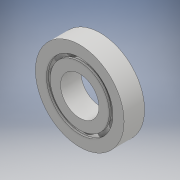
# Autodesk Inventor part: Подшипник 1
Saved by Autodesk Inventor 2018.1 (Build 221171000, 171)
## iProperties
Created: 2018-06-08
Part Number: Подшипник 1
Material: Типовые
Document SubType Name: Modeling
Designer: Dmitry
Density: 1 g/cm^3
Appearance: По умолчанию
Author: Dmitry
Autodesk Inventor part; units mm, degrees
ref_plane "YZ Plane" through (0, 0, 0) normal (1, 0, 0) x (0, 1, 0)
ref_plane "XZ Plane" through (0, 0, 0) normal (0, 1, 0) x (-1, 0, 0)
ref_plane "XY Plane" through (0, 0, 0) normal (0, 0, 1) x (1, 0, 0)
sketch "Эскиз1" plane through (0, 0, 0) normal (0, 0, 1) x (1, 0, 0)
  line L0 (26, 0) -> (26, 27.7778)
  line L1 (26, 27.7778) -> (40, 27.7778)
  line L2 (40, 27.7778) -> (40, 25)
  line L3 (40, 2.7778) -> (40, 0)
  line L4 (40, 0) -> (26, 0)
  arc A0 (40, 25) -> (40, 2.7778) centre (46.2467, 13.8889) ccw
  line L5 (60, 0) -> (60, 27.7778)
  line L6 (60, 27.7778) -> (45, 27.7778)
  line L7 (45, 27.7778) -> (45, 25)
  line L8 (45, 2.7778) -> (45, 0)
  line L9 (45, 0) -> (60, 0)
  arc A1 (45, 2.7778) -> (45, 25) centre (40.5195, 13.8889) ccw
  line L10 (0, -5.5556) -> (0, 33.3333) projected
  constraints: 20 end point, 4 point on circle, 2 centre point
revolve "Вращение1" add sketch "Эскиз1" angle 360 about axis through (0, -10, 0) along (0, 1, 0)
sketch "Эскиз2" plane through (0, 0, 0) normal (1, 0, 0) x (0, 1, 0)
  line L0 (13.8889, 50.6) -> (13.8889, 35.4)
  arc A0 (13.8889, 35.4) -> (13.8889, 50.6) centre (14.59, 43) ccw
  constraints: 2 end point, 2 point on circle, 1 centre point
revolve "Вращение2" add sketch "Эскиз2" angle 360 about axis through (0, 13.8889, 50.6) along (0, 0, -1) separate body
pattern_circular "Круговой массив1" count 12 over 360 about axis through (0, -10, 0) along (0, 1, 0) of "Вращение2" bodies 2
